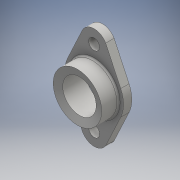
# Autodesk Inventor part: パッキン押え
Saved by Autodesk Inventor 2016 SP1 (Build 200210100, 210)
## iProperties
Created: 2016-12-20
Part Number: パッキン押え
Material: 一般
Document SubType Name: Modeling
Designer: p_admin
Density: 1 g/cm^3
Appearance: 既定
Author: p_admin
Autodesk Inventor part; units mm, degrees
ref_plane "YZ Plane" through (0, 0, 0) normal (1, 0, 0) x (0, 1, 0)
ref_plane "XZ Plane" through (0, 0, 0) normal (0, 1, 0) x (-1, 0, 0)
ref_plane "XY Plane" through (0, 0, 0) normal (0, 0, 1) x (1, 0, 0)
sketch "スケッチ1" plane through (0, 0, 0) normal (0, 1, 0) x (-1, 0, 0)
  circle A0 centre (0, 0) radius 20
  circle A1 centre (0, 0) radius 29
  arc A2 (31.7208, -14.7916) -> (31.7208, 14.7916) centre (0, 0) ccw
  line L0 (0, 0) -> (31.7208, 14.7916) construction
  line L1 (0, 0) -> (35, 0) construction
  line L2 (0, 0) -> (31.7208, -14.7916) construction
  arc A3 (-31.7129, 14.8084) -> (-31.7208, -14.7915) centre (0, 0) ccw
  circle A4 centre (0.0475, 45) radius 6.5
  circle A5 centre (-0.0487, -45) radius 6.5
  arc A6 (13.9039, 53) -> (-13.8089, 53) centre (0.0475, 45) ccw
  line L3 (0.0475, 45) -> (13.9039, 53) construction
  line L4 (0.0475, 45) -> (16.0475, 45) construction
  line L5 (0.0475, 45) -> (-13.8089, 53) construction
  arc A7 (-13.8991, -53.0102) -> (13.8137, -52.9897) centre (-0.0487, -45) ccw
  line L6 (-0.0487, -45) -> (-13.8991, -53.0102) construction
  line L7 (-0.0487, -45) -> (13.8137, -52.9897) construction
  line L8 (13.9039, 53) -> (31.7208, 14.7916)
  line L9 (-13.8089, 53) -> (-31.7129, 14.8084)
  line L10 (-31.7208, -14.7915) -> (-13.8991, -53.0102)
  line L11 (13.8137, -52.9897) -> (31.7208, -14.7916)
  dimension "d0" = 40
  dimension "d1" = 58
  dimension "d2" = 35
  dimension "d3" = 25
  dimension "d4" = 50
  dimension "d5" = 35
  dimension "d6" = 13
  dimension "d7" = 13
  dimension "d8" = 45
  dimension "d9" = 45
  dimension "d10" = 16
  dimension "d11" = 30
  dimension "d12" = 120
  dimension "d13" = 16
  dimension "d14" = 120
  constraints: 24 end point, 8 centre point, 8 point on circle, 6 coincident, 2 equal length, 2 horizontal, 2 parallel, 1 concentric, 1 perpendicular
  measures "d0" diameter of A0
  measures "d1" diameter of A1
  measures "d2" radius of A2
  measures "d3" angle of L1 L0
  measures "d4" angle of L2 L0
  measures "d5" radius of A3
  measures "d6" diameter of A4
  measures "d7" diameter of A5
  measures "d8" distance of point (0, 0) A4.centre
  measures "d9" distance of point (0, 0) A5.centre
  measures "d10" radius of A6
  measures "d11" angle of L4 L3
  measures "d12" angle of L3 L5
  measures "d13" radius of A7
  measures "d14" angle of L6 L7
extrude "押し出し1" add sketch "スケッチ1" along normal blind 10 contours A1 | L11 A7 L10 A3 L9 A6 L8 A2
sketch "スケッチ2" plane through (0, 0, 0) normal (0, -1, 0) x (1, 0, 0)
  circle A0 centre (0, 0) radius 29
  circle A1 centre (0, 0) radius 20
  dimension "d17" = 58
  constraints: 2 centre point, 2 coincident
  measures "d17" diameter of A0
extrude "押し出し2" add sketch "スケッチ2" along normal blind 20
chamfer "面取り1" distance 9 angle 15 1 edges at (-20, -20, 0) measured on face at (25.5254, -20, -3.9088)
fillet "フィレット1" radius 2 1 edges at (-29, 0, 0)
